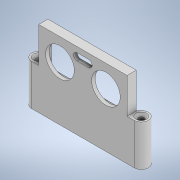
# Autodesk Inventor part: Крепление ультрасоника
Saved by Autodesk Inventor 2020 (Build 240168000, 168)
## iProperties
Created: 2021-05-10
Part Number: Крепление ультрасоника
Material: Типовые
Document SubType Name: Modeling
Designer: Антон
Density: 1 g/cm^3
Appearance: По умолчанию
Author: Антон
Autodesk Inventor part; units mm, degrees
ref_plane "YZ Plane" through (0, 0, 0) normal (1, 0, 0) x (0, 1, 0)
ref_plane "XZ Plane" through (0, 0, 0) normal (0, 1, 0) x (-1, 0, 0)
ref_plane "XY Plane" through (0, 0, 0) normal (0, 0, 1) x (1, 0, 0)
sketch "Эскиз1" plane through (0, 0, 0) normal (0, 0, 1) x (1, 0, 0)
  line L0 (0, 0) -> (50, 0)
  line L1 (50, 0) -> (50, 25)
  line L2 (50, 25) -> (0, 25)
  line L3 (0, 25) -> (0, 0)
  dimension "d0" = 50
  dimension "d1" = 25
  constraints: 8 end point, 2 parallel, 1 horizontal, 1 perpendicular
  measures "d0" distance of L2.end L1.end
  measures "d1" distance of L1.end L0.end
extrude "Выдавливание1" add sketch "Эскиз1" along normal blind 5.2
shell "Оболочка1" thickness 2 removed faces 1 at (16.6667, 16.6667, 0)
sketch "Эскиз2" plane through (0, 0, 5.2) normal (0, 0, 1) x (1, 0, 0)
  line L0 (50, 25) -> (0, 25) projected
  line L1 (25, 25) -> (25, 0)
  line L2 (0, 0) -> (50, 0) projected
  line L3 (25, 12.5) -> (12, 12.5)
  line L4 (0, 25) -> (0, 0) projected
  circle A0 centre (12, 12.5) radius 8.1
  circle A1 centre (38, 12.5) radius 8.1
  line L5 (25, 25) -> (25, 20)
  line L6 (21.75, 20) -> (28.25, 20) construction
  line L7 (21.75, 18) -> (28.25, 18)
  line L8 (28.25, 22) -> (21.75, 22)
  arc A2 (21.75, 22) -> (21.75, 18) centre (21.75, 20) ccw
  arc A3 (28.25, 18) -> (28.25, 22) centre (28.25, 20) ccw
  point P0 (25, 18)
  point P1 (25, 22)
  dimension "d5" = 13
  dimension "d6" = 16.2
  dimension "d9" = 5
  dimension "d10" = 3.25
  dimension "d11" = 4
  constraints: 14 end point, 4 centre point, 4 midpoint, 4 point on circle, 4 tangent, 1 coincident, 1 horizontal, 1 parallel, 1 perpendicular, 1 point on line, 1 symmetric about line, 1 other
  measures "d5" distance of L3.start L3.end
  measures "d6" diameter of A0
  measures "d9" distance of L1.start L5.end
  measures "d10" distance of L5.end L6.end
  measures "d11" diameter of A3
extrude "Выдавливание2" cut sketch "Эскиз2" against normal through all contours L8 A3 L7 L1 | L1 L7 A2 L8 | A0 | A1
sketch "Эскиз5" plane through (48, 23, 3.2) normal (0, 0, -1) x (-1, 0, 0)
  line L0 (0, 0) -> (1.05, 0)
  line L1 (0, 0) -> (46, 0) projected
  line L2 (1.05, 0) -> (1.05, -1.05)
  circle A0 centre (1.05, -1.05) radius 1.05
  line L3 (2.1, -2.1) -> (0, -2.1)
  line L4 (0, -2.1) -> (0, 0)
  line L5 (0, 0) -> (2.1, 0)
  line L6 (2.1, 0) -> (2.1, -2.1)
  line L7 (2.1, -2.1) -> (0, 0) construction
  line L8 (0, -2.1) -> (2.1, 0) construction
  point P0 (48, -23)
  point P1 (1.05, -2.1)
  point P2 (2.1, -1.05)
  dimension "d17" = 1.05
  dimension "d18" = 1.05
  constraints: 16 end point, 2 midpoint, 2 parallel, 1 coincident, 1 horizontal, 1 perpendicular, 1 point on line, 1 vertical, 3 other
  measures "d17" distance of L0.start L0.end
  measures "d18" distance of L0.end L2.end
extrude "Выдавливание4" add sketch "Эскиз5" along normal blind 1 contours L0 A0 L4 | L1 L6 A0 | A0 | A0 L3 L4
ref_plane "РабПлоскость1" through (25, 2, 0) normal (1, 0, 0) x (0, 0, -1)
ref_plane "РабПлоскость2" through (2, 12.5, 0) normal (0, -1, 0) x (1, 0, 0)
mirror "Зеркальное отражение1" about plane through (2, 12.5, 0) normal (0, -1, 0) of "Выдавливание4"
mirror "Зеркальное отражение2" about plane through (25, 2, 0) normal (1, 0, 0) of "Выдавливание4", "Зеркальное отражение1"
sketch "Эскиз7" plane through (0, 0, 0) normal (0, -1, 0) x (1, 0, 0)
  line L0 (0, 0) -> (50, 0) projected
  line L1 (50, 0) -> (50, 5.2) projected
  line L2 (0, 5.2) -> (50, 5.2) projected
  line L3 (0, 0) -> (0, 5.2) projected
  line L4 (50, 5.2) -> (0, 5.2) projected
  line L5 (50, 5.2) -> (58, 5.2)
  line L6 (58, 5.2) -> (58, -2.8)
  line L7 (58, -2.8) -> (50, -2.8)
  line L8 (50, -2.8) -> (50, 5.2)
  point P0 (50, 0)
  dimension "d24" = 8
  dimension "d25" = 8
  constraints: 8 end point, 2 parallel, 1 collinear, 1 horizontal, 1 perpendicular, 1 point on line
  measures "d24" distance of L6.end L7.end
  measures "d25" distance of L5.end L6.end
extrude "Выдавливание6" add sketch "Эскиз7" against normal blind 5 contours L1 L5 L6 L7 L8
sketch "Эскиз8" plane through (47.1, 5, 0) normal (0, 1, 0) x (-1, 0, 0)
  line L0 (-10.9, 5.2) -> (-10.9, -2.8) projected
  line L1 (-10.9, 1.2) -> (-2.9, 1.2)
  line L2 (-10.9, -2.8) -> (-2.9, -2.8) projected
  line L3 (-2.9, -2.8) -> (-2.9, 0) projected
  line L4 (-2.9, 5.2) -> (-2.9, 0) projected
  line L5 (-2.9, 5.2) -> (-10.9, 5.2) projected
  line L6 (-10.9, 5.2) -> (-10.9, -2.8) projected
  point P0 (47.1, 0)
  point P1 (-10, 5.2)
  point P2 (-10, -2.8)
  point P3 (-6.9, 1.2)
  constraints: 2 end point, 1 horizontal, 1 midpoint, 1 point on line, 2 other
hole "Отверстие1" at (54, 5, 1.2) direction (0, -1, 0) diameter 3.2 end through all countersink diameter 6 countersink angle 90
fillet "Сопряжение1" radius 4 2 edges at (58, 2.5, -2.8) (58, 2.5, 5.2)
fillet "Сопряжение1" radius 4.3 1 edges at (50, 2.5, -2.8)
ref_plane "РабПлоскость3" through (25, 25, 5.2) normal (1, 0, 0) x (0, 0, -1)
mirror "Зеркальное отражение3" about plane through (25, 25, 5.2) normal (1, 0, 0) of "Сопряжение1", "Отверстие1", "Выдавливание6"
sketch "Эскиз9" plane through (54, 0, 1.2) normal (0, -1, 0) x (1, 0, 0)
  arc A0 (-58, -4) -> (-54, -1.2) centre (-58.0299, 0.2999) ccw projected
  line L0 (-54, -1.2) -> (-4, -1.2) projected
  arc A1 (-4, -1.2) -> (0, -4) centre (0.0299, 0.2999) ccw projected
  arc A2 (0, -4) -> (0, 4) centre (0, 0) ccw projected
  line L1 (-58, 4) -> (0, 4) projected
  arc A3 (-58, 4) -> (-58, -4) centre (-58, 0) ccw projected
  circle A4 centre (0, 0) radius 1.6 projected
  circle A5 centre (-58, 0) radius 1.6 projected
extrude "Выдавливание7" add sketch "Эскиз9" along normal blind 18.25
ref_plane "РабПлоскость4" through (25, 25, 5.2) normal (1, 0, 0) x (0, 0, -1)
